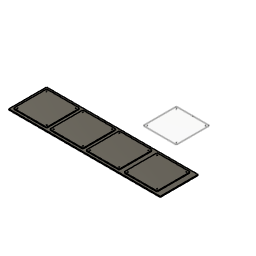
AprilTagStandv8 (Autodesk Fusion 360 archive; units mm, degrees)
design "AprilTagPlate"
Autodesk Fusion 360 part; units mm, degrees
sketch "Sketch1" plane through (0, 0, 0) normal (0, 0, 1) x (1, 0, 0)
  line L0 (6.35, 0) -> (260.35, 0)
  line L1 (266.7, 6.35) -> (266.7, 260.35)
  line L2 (0, 260.35) -> (0, 6.35)
  arc A0 (6.35, 266.7) -> (0, 260.35) centre (6.35, 260.35) ccw
  arc A1 (266.7, 260.35) -> (260.35, 266.7) centre (260.35, 260.35) ccw
  arc A2 (260.35, 0) -> (266.7, 6.35) centre (260.35, 6.35) ccw
  arc A3 (0, 6.35) -> (6.35, 0) centre (6.35, 6.35) ccw
  line L3 (0, 16.002) -> (266.7, 16.002) construction
  line L4 (16.002, 0) -> (16.002, 266.7) construction
  line L5 (0, 250.952) -> (266.7, 250.952) construction
  line L6 (250.952, 0) -> (250.952, 266.7) construction
  circle A4 centre (16.002, 250.952) radius 3.429
  circle A5 centre (250.952, 250.952) radius 3.429
  circle A6 centre (250.952, 16.002) radius 3.429
  circle A7 centre (16.002, 16.002) radius 3.429
  arc A8 (131.7835, 266.1786) -> (131.0605, 266.7) centre (131.0605, 265.938) ccw
  arc A9 (135.6395, 266.7) -> (134.9165, 266.1786) centre (135.6395, 265.938) ccw
  arc A10 (131.7835, 266.1786) -> (134.9165, 266.1786) centre (133.35, 266.7) ccw
  line L7 (260.35, 266.7) -> (135.6395, 266.7)
  line L8 (131.0605, 266.7) -> (6.35, 266.7)
  line L9 (237.998, 0) -> (237.998, 16.002)
  line L10 (250.698, 28.702) -> (266.7, 28.702)
  arc A11 (250.698, 28.702) -> (237.998, 16.002) centre (250.698, 16.002) ccw
  line L11 (28.702, 0) -> (28.702, 16.002)
  line L12 (16.002, 28.702) -> (0, 28.702)
  line L13 (28.702, 266.7) -> (28.702, 250.698)
  line L14 (16.002, 237.998) -> (0, 237.998)
  line L15 (237.998, 266.7) -> (237.998, 250.698)
  line L16 (250.698, 237.998) -> (266.7, 237.998)
  arc A12 (28.702, 16.002) -> (16.002, 28.702) centre (16.002, 16.002) ccw
  arc A13 (16.002, 237.998) -> (28.702, 250.698) centre (16.002, 250.698) ccw
  arc A14 (237.998, 250.698) -> (250.698, 237.998) centre (250.698, 250.698) ccw
  point P0 (266.7, 0)
  point P1 (0, 266.7)
  dimension "d1" = 266.7
  dimension "d2" = 266.7
  dimension "d3" = 6.35
  dimension "d4" = 16.002
  dimension "d5" = 250.952
  dimension "d6" = 16.002
  dimension "d7" = 250.952
  dimension "d8" = 6.858
  dimension "d9" = 3.302
  dimension "d10" = 1.524
  dimension "d11" = 1.524
  dimension "d12" = 28.702
  dimension "d13" = 28.702
  dimension "d14" = 12.7
  dimension "d15" = 12.7
  dimension "d16" = 28.702
  dimension "d17" = 28.702
  dimension "d18" = 28.702
  dimension "d19" = 28.702
  dimension "d20" = 28.702
  dimension "d21" = 28.702
  constraint horizontal L0
  constraint vertical L1
  constraint horizontal L7
  constraint vertical L2
  constraint coincident P1 L7
  constraint coincident P1 L2
  constraint tangent A0 L7
  constraint tangent L2 A0
  constraint tangent L1 A1
  constraint tangent A1 L7
  constraint equal A0 A1
  constraint coincident P0 L0
  constraint coincident P0 L1
  constraint tangent L0 A2
  constraint tangent L1 A2
  constraint equal A0 A2
  constraint coincident origin L0
  constraint coincident origin L2
  constraint tangent L0 A3
  constraint tangent L2 A3
  constraint equal A0 A3
  constraint coincident L2 L3.start
  constraint coincident L1 L3.end
  constraint perpendicular L1 L3
  constraint coincident L0 L4.start
  constraint coincident L4.end L7
  constraint perpendicular L4 L7
  constraint coincident L2 L5.start
  constraint coincident L1 L5.end
  constraint perpendicular L1 L5
  constraint coincident L0 L6.start
  constraint coincident L6.end L7
  constraint perpendicular L6 L7
  constraint coincident L4 A4.centre
  constraint coincident L5 A4.centre
  constraint coincident L5 A5.centre
  constraint coincident L6 A5.centre
  constraint coincident L6 A6.centre
  constraint coincident L3 A6.centre
  constraint coincident L3 A7.centre
  constraint coincident L4 A7.centre
  constraint equal A4 A7
  constraint equal A4 A5
  constraint equal A4 A6
  constraint tangent A8 L7
  constraint tangent A9 L7
  constraint tangent A9 A10
  constraint tangent A8 A10
  constraint coincident A8.end L7
  constraint collinear L7 L8
  constraint coincident A10.centre L7
  constraint coincident L0 L9.start
  constraint perpendicular L3 L9
  constraint coincident L1 L10.end
  constraint perpendicular L1 L10
  constraint tangent L9 A11
  constraint tangent L10 A11
  constraint coincident L0 L11.start
  constraint perpendicular L0 L11
  constraint coincident L2 L12.end
  constraint perpendicular L2 L12
  constraint coincident L8 L13.start
  constraint perpendicular L5 L13
  constraint coincident L2 L14.end
  constraint perpendicular L2 L14
  constraint coincident L7 L15.start
  constraint perpendicular L7 L15
  constraint coincident L1 L16.end
  constraint perpendicular L1 L16
  constraint tangent L11 A12
  constraint tangent L12 A12
  constraint tangent L13 A13
  constraint tangent L14 A13
  constraint equal A12 A13
  constraint tangent L15 A14
  constraint tangent L16 A14
  constraint equal A12 A14
  measures "d1" distance of origin P0
  measures "d2" distance of origin P1
  measures "d3" radius of A0
  measures "d4" distance of L0 L3
  measures "d5" distance of L0 L5
  measures "d6" distance of L2 L4
  measures "d7" distance of L2 L6
  measures "d8" diameter of A4
  measures "d9" diameter of A10
  measures "d10" diameter of A9
  measures "d11" diameter of A8
  measures "d12" distance of L0 L10
  measures "d13" distance of L1 L9
  measures "d14" radius of A11
  measures "d15" radius of A12
  measures "d16" distance of L0 L12
  measures "d17" distance of L2 L11
  measures "d18" distance of L2 L13
  measures "d19" distance of L8 L14
  measures "d20" distance of L1 L15
  measures "d21" distance of L7 L16
extrude "Extrude1" add sketch "Sketch1" against normal blind 5.4102 makes body 1
copy_body "Body->Comp1" bodies 1 removing the originals makes body 2 in component "backer"
sketch "Sketch2" plane through (0, 0, 0) normal (0, 0, 1) x (1, 0, 0)
  line L0 (-648.4709, -129.141) -> (570.7291, -129.141)
  line L1 (570.7291, -129.141) -> (570.7291, -433.941)
  line L2 (570.7291, -433.941) -> (-648.4709, -433.941)
  line L3 (-648.4709, -433.941) -> (-648.4709, -129.141)
  dimension "d24" = 1219.2
  dimension "d25" = 304.8
  constraint horizontal L0
  constraint vertical L1
  constraint horizontal L2
  constraint vertical L3
  measures "d24" distance of L0.start L0.end
  measures "d25" distance of L0.start L2.end
extrude "Extrude2" add sketch "Sketch2" along normal blind 6.35 separate body makes body 3
copy_body "Body->Comp2" bodies 3 removing the originals makes body 4 in component "cnc"
component "backer" placed x (1, 0, 0) y (0, 1, 0) z (0, 0, 1) at (0, 0, 0)
component "cnc" placed x (1, 0, 0) y (0, 1, 0) z (0, 0, 1) at (0, 0, 0)
component "backer" placed x (1, 0, 0) y (0, -1, 0) z (0, 0, -1) at (-337.3209, -148.191, 6.35) in component "cnc"
component "backer" placed x (1, 0, 0) y (0, -1, 0) z (0, 0, -1) at (259.5791, -148.191, 6.35) in component "cnc"
component "backer" placed x (1, 0, 0) y (0, -1, 0) z (0, 0, -1) at (-45.2209, -148.191, 6.35) in component "cnc"
component "backer" placed x (1, 0, 0) y (0, -1, 0) z (0, 0, -1) at (-629.4209, -148.191, 6.35) in component "cnc"
equation "d6 = d4"
equation "d7 = d5"
equation "d13 = d12"
equation "d16 = d12"
equation "d17 = d13"
equation "d18 = d16"
equation "d19 = d18"
equation "d20 = d18"
equation "d21 = d20"
